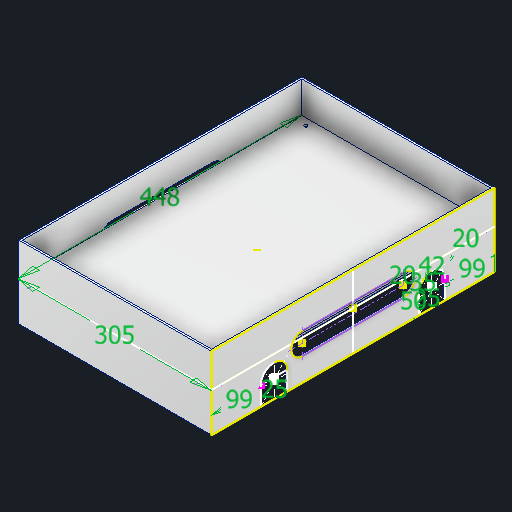
# Autodesk Inventor part: AMR_Top_Basket
Saved by Autodesk Inventor 2026.2 (Build 302298010, 298A)
## iProperties
Created: 2026-03-25
Part Number: AMR_Top_Basket
Material: Aluminum 6061
Document SubType Name: Modeling
Designer: Srishanth Dhondy
Density: 2.7 g/cm^3
Appearance: Aluminum - Flat
Mass: 2257.86 g
Surface Area: 5680.06 cm^2
Volume: 836.244 cm^3
Author: Srishanth Dhondy
Autodesk Inventor part; units mm, degrees
ref_plane "YZ Plane" through (0, 0, 0) normal (1, 0, 0) x (0, 1, 0)
ref_plane "XZ Plane" through (0, 0, 0) normal (0, 1, 0) x (-1, 0, 0)
sketch "Sketch1" plane through (0, 0, 0) normal (0, 1, 0) x (-1, 0, 0)
  line L0 (-152.5, -224) -> (152.5, -224)
  line L1 (152.5, -224) -> (152.5, 224)
  line L2 (152.5, 224) -> (-152.5, 224)
  line L3 (-152.5, 224) -> (-152.5, -224)
  line L4 (-152.5, -224) -> (152.5, 224) construction
  line L5 (152.5, -224) -> (-152.5, 224) construction
  point P0 (0, 0)
  point P1 (132, 210)
  point P2 (-132, -210)
  point P3 (132, -210)
  point P4 (-132, 210)
  dimension "d0" = 305
  dimension "d1" = 448
  constraints: 12 end point, 2 midpoint, 2 parallel, 1 horizontal, 1 perpendicular
  measures "d0" distance of L2.end L1.end
  measures "d1" distance of L1.end L0.end
extrude "Extrusion1" add sketch "Sketch1" along normal blind 3
sketch "Sketch2" plane through (0, 3, 0) normal (0, 1, 0) x (1, 0, 0)
  line L0 (-152.5, 224) -> (-152.5, -224) projected
  line L1 (-152.5, -224) -> (152.5, -224) projected
  line L2 (152.5, -224) -> (152.5, 224) projected
  line L3 (152.5, 224) -> (-152.5, 224) projected
  line L4 (-152.5, 224) -> (-152.5, -224) projected
  line L5 (-152.5, -224) -> (152.5, -224) projected
  line L6 (152.5, -224) -> (152.5, 224) projected
  line L7 (152.5, 224) -> (-152.5, 224) projected
  line L8 (-149.5, -221) -> (-149.5, 221)
  line L9 (-149.5, 221) -> (149.5, 221)
  line L10 (149.5, 221) -> (149.5, -221)
  line L11 (149.5, -221) -> (-149.5, -221)
  point P0 (0, 0)
  dimension "d4" = 3
  constraints: 8 end point, 3 other
  measures "d4" distance between parallel lines of L0 L8
extrude "Extrusion2" add sketch "Sketch2" along normal blind 50 and the other way blind 65
hole "Hole1" at (132, 0, -210) at (132, 0, 210) at (-132, 0, 210) at (-132, 0, -210) direction (0, 1, 0) diameter 5 end through all
sketch "Sketch3" plane through (152.5, -62, -224) normal (1, 0, 0) x (0, 0, -1)
  line L0 (0, 0) -> (0, 115) projected
  line L1 (-448, 115) -> (0, 115) projected
  line L2 (-448, 0) -> (-448, 115) projected
  line L3 (0, 0) -> (-448, 0) projected
  point P0 (-224, 62)
sketch "Sketch4" plane through (152.5, -62, -224) normal (1, 0, 0) x (0, 0, -1)
  line L0 (0, 0) -> (0, 115) projected
  line L1 (-448, 115) -> (0, 115) projected
  line L2 (-448, 0) -> (-448, 115) projected
  line L3 (0, 0) -> (-448, 0) projected
  point P0 (-224, 62)
sketch "Sketch5" plane through (152.5, -62, -224) normal (1, 0, 0) x (0, 0, -1)
  line L0 (0, 0) -> (0, 115) projected
  line L1 (-448, 115) -> (0, 115) projected
  line L2 (-448, 0) -> (-448, 115) projected
  line L3 (0, 0) -> (-448, 0) projected
  line L4 (0, 0) -> (-448, 0) projected
  point P0 (-224, 62)
  point P1 (-224, 62)
  point P2 (-99, 25)
  dimension "d16" = 99
  dimension "d17" = 25
  measures "d16" horizontal distance of L0.start point (-99, 25)
  measures "d17" distance from line of L3 point (-99, 25)
sketch "Sketch6" plane through (152.5, -62, -224) normal (1, 0, 0) x (0, 0, -1)
  line L0 (0, 0) -> (-448, 0) projected
  line L1 (-445, 115) -> (-3, 115) projected
  line L2 (-224, 115) -> (-224, 0)
  line L3 (-78, 0) -> (-120, 0)
  line L4 (-120, 0) -> (-120, 30)
  line L5 (-100, 50) -> (-98, 50)
  line L6 (-78, 30) -> (-78, 0)
  line L7 (-78, 0) -> (-120, 50) construction
  line L8 (-120, 0) -> (-78, 50) construction
  line L9 (-448, 0) -> (-448, 115) projected
  arc A0 (-100, 50) -> (-120, 30) centre (-100, 30) ccw
  arc A1 (-78, 30) -> (-98, 50) centre (-98, 30) ccw
  line L10 (-328, 0) -> (-328, 30)
  line L11 (-370, 30) -> (-370, 0)
  line L12 (-370, 0) -> (-328, 50) construction
  line L13 (-328, 0) -> (-370, 50) construction
  arc A2 (-328, 30) -> (-348, 50) centre (-348, 30) ccw
  arc A3 (-350, 50) -> (-370, 30) centre (-350, 30) ccw
  line L14 (-304.3108, 54.0001) -> (-144.3108, 54.0001) construction
  line L15 (-445, 62) -> (-3, 62) projected
  line L16 (-304.3108, 36.5001) -> (-144.3108, 36.5001)
  line L17 (-144.3108, 71.5001) -> (-304.3108, 71.5001)
  arc A4 (-304.3108, 71.5001) -> (-304.3108, 36.5001) centre (-304.3108, 54.0001) ccw
  arc A5 (-144.3108, 36.5001) -> (-144.3108, 71.5001) centre (-144.3108, 54.0001) ccw
  line L18 (-370, 0) -> (-328, 0)
  line L19 (-328, 0) -> (-328, 30)
  line L20 (-328, 30) -> (-370, 30)
  line L21 (-370, 30) -> (-370, 0)
  line L22 (-350, 50) -> (-348, 50)
  point P0 (-224, 62)
  point P1 (-99, 25)
  point P2 (-99, 25)
  point P3 (-99, 25)
  point P4 (-120, 0)
  point P5 (-78, 0)
  point P6 (-349, 25)
  point P7 (-349, 25)
  point P8 (-99, 50)
  point P9 (-349, 50)
  point P10 (-370, 0)
  point P11 (-328, 0)
  point P12 (-224.3108, 54.0001)
  point P13 (-304.3108, 54.0001)
  dimension "d18" = 42
  dimension "d19" = 50
  dimension "d26" = 20
  dimension "d27" = 20
  dimension "d28" = 99
  dimension "d29" = 25
  dimension "d32" = 35
  constraints: 40 end point, 12 point on circle, 11 symmetric about line, 8 tangent, 6 centre point, 6 midpoint, 6 parallel, 6 point on line, 3 horizontal, 2 coincident, 2 perpendicular, 2 other
  measures "d18" distance of L7.end L8.end
  measures "d19" distance of L3.end L7.end
  measures "d26" radius of A0
  measures "d27" radius of A1
  measures "d28" distance from line of L9 point (-349, 25)
  measures "d29" distance from line of point (-349, 25) L0
  measures "d32" diameter of A5
extrude "Extrusion3" cut sketch "Sketch6" against normal through all contours L0 L4 A0 L5 A1 L6
extrude "Extrusion4" cut sketch "Sketch6" against normal through all contours L0 L11 L20 L10 | L20 A3 L22 A2
extrude "Extrusion5" cut sketch "Sketch6" against normal blind 3 contours L16 A4 L15 L2 | L2 L15 A5 L16 | L15 A4 L17 L2 | L2 L17 A5 L15
sketch "Sketch7" plane through (152.5, -62, -224) normal (1, 0, 0) x (0, 0, -1)
  arc A0 (-144.3108, 36.5001) -> (-144.3108, 71.5001) centre (-144.3108, 54.0001) ccw projected
  line L0 (-144.3108, 36.5001) -> (-304.3108, 36.5001) projected
  arc A1 (-304.3108, 71.5001) -> (-304.3108, 36.5001) centre (-304.3108, 54.0001) ccw projected
  line L1 (-304.3108, 71.5001) -> (-144.3108, 71.5001) projected
  line L2 (-370, 0) -> (-370, 30) projected
  arc A2 (-328, 30) -> (-348, 50) centre (-348, 30) ccw projected
  line L3 (-328, 30) -> (-328, 0) projected
  line L4 (-120, 0) -> (-328, 0) projected
  line L5 (-120, 0) -> (-120, 30) projected
  arc A3 (-100, 50) -> (-120, 30) centre (-100, 30) ccw projected
  line L6 (-78, 30) -> (-78, 0) projected
  line L7 (0, 0) -> (-78, 0) projected
  line L8 (0, 0) -> (0, 115) projected
  line L9 (-448, 115) -> (0, 115) projected
  line L10 (-448, 0) -> (-448, 115) projected
  line L11 (-370, 0) -> (-448, 0) projected
  point P0 (-369, 30)
  point P1 (-79, 30)
  point P2 (-224, 62)
  constraints: 2 other
ref_plane "Work Plane2" through (0, -62, -224) normal (1, 0, 0) x (0, 0, -1)
sketch "Sketch8" plane through (152.5, -62, -224) normal (1, 0, 0) x (0, 0, -1)
  arc A0 (-144.3108, 36.5001) -> (-144.3108, 71.5001) centre (-144.3108, 54.0001) ccw projected
  line L0 (-144.3108, 36.5001) -> (-304.3108, 36.5001) projected
  arc A1 (-304.3108, 71.5001) -> (-304.3108, 36.5001) centre (-304.3108, 54.0001) ccw projected
  line L1 (-304.3108, 71.5001) -> (-144.3108, 71.5001) projected
  line L2 (-370, 0) -> (-370, 30) projected
  arc A2 (-328, 30) -> (-348, 50) centre (-348, 30) ccw projected
  line L3 (-328, 30) -> (-328, 0) projected
  line L4 (-120, 0) -> (-328, 0) projected
  line L5 (-120, 0) -> (-120, 30) projected
  arc A3 (-100, 50) -> (-120, 30) centre (-100, 30) ccw projected
  line L6 (-78, 30) -> (-78, 0) projected
  line L7 (0, 0) -> (-78, 0) projected
  line L8 (0, 0) -> (0, 115) projected
  line L9 (-448, 115) -> (0, 115) projected
  line L10 (-448, 0) -> (-448, 115) projected
  line L11 (-370, 0) -> (-448, 0) projected
  point P0 (-369, 30)
  point P1 (-79, 30)
  point P2 (-224, 62)
  constraints: 2 other
mirror "Mirror1" about plane through (0, -62, -224) normal (1, 0, 0) of "Extrusion5"
body "Solid1"
